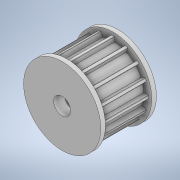
# Autodesk Inventor part: zahnrad2
Saved by Autodesk Inventor 2021 (Build 250183000, 183)
## iProperties
Created: 2021-08-20
Part Number: zahnrad2
Material: Generisch
Document SubType Name: Modeling
Designer: stroh
Density: 1 g/cm^3
Appearance: Vorgabe
Author: stroh
Autodesk Inventor part; units mm, degrees
ref_plane "YZ Plane" through (0, 0, 0) normal (1, 0, 0) x (0, 1, 0)
ref_plane "XZ Plane" through (0, 0, 0) normal (0, 1, 0) x (-1, 0, 0)
ref_plane "XY Plane" through (0, 0, 0) normal (0, 0, 1) x (1, 0, 0)
sketch "Skizze1" plane through (0, 0, 0) normal (0, 0, 1) x (1, 0, 0)
  circle A0 centre (0, 0) radius 9.99
  dimension "d0" = 19.98
  constraints: 1 centre point, 1 coincident
  measures "d0" diameter of A0
extrude "Extrusion1" add sketch "Skizze1" along normal blind 15
sketch "Skizze2" plane through (0, 0, 15) normal (0, 0, 1) x (1, 0, 0)
  circle A0 centre (0, 0) radius 9.99 projected
  line L0 (-0.5, 9.9775) -> (0.5, 9.9775)
  line L1 (-0.5, 9.9775) -> (-0.5177, 11.3774)
  line L2 (0.4823, 11.3774) -> (0.5, 9.9775)
  line L3 (-0.5177, 11.3774) -> (-0.419, 11.4786)
  line L4 (0.381, 11.4786) -> (0.4823, 11.3774)
  line L5 (-0.419, 11.4786) -> (0.381, 11.4786)
  line L6 (-4.2802, 9.0266) -> (-4.8322, 10.3132)
  line L7 (-4.8322, 10.3132) -> (-4.7798, 10.4445)
  line L8 (-4.7798, 10.4445) -> (-4.0407, 10.7507)
  line L9 (-4.0407, 10.7507) -> (-3.9084, 10.6959)
  line L10 (-3.9084, 10.6959) -> (-3.3563, 9.4093)
  line L11 (-4.2802, 9.0266) -> (-3.3563, 9.4093)
  line L12 (-7.4087, 6.7016) -> (-8.4111, 7.6789)
  line L13 (-8.4111, 7.6789) -> (-8.4129, 7.8203)
  line L14 (-8.4129, 7.8203) -> (-7.8472, 8.386)
  line L15 (-7.8472, 8.386) -> (-7.704, 8.386)
  line L16 (-7.704, 8.386) -> (-6.7016, 7.4087)
  line L17 (-7.4087, 6.7016) -> (-6.7016, 7.4087)
  line L18 (-9.4093, 3.3563) -> (-10.7094, 3.8756)
  line L19 (-10.7094, 3.8756) -> (-10.7652, 4.0056)
  line L20 (-10.7652, 4.0056) -> (-10.4591, 4.7447)
  line L21 (-10.4591, 4.7447) -> (-10.3268, 4.7995)
  line L22 (-10.3268, 4.7995) -> (-9.0266, 4.2802)
  line L23 (-9.4093, 3.3563) -> (-9.0266, 4.2802)
  line L24 (-9.9775, -0.5) -> (-11.3774, -0.5177)
  line L25 (-11.3774, -0.5177) -> (-11.4786, -0.419)
  line L26 (-11.4786, -0.419) -> (-11.4786, 0.381)
  line L27 (-11.4786, 0.381) -> (-11.3774, 0.4823)
  line L28 (-11.3774, 0.4823) -> (-9.9775, 0.5)
  line L29 (-9.9775, -0.5) -> (-9.9775, 0.5)
  line L30 (-9.0266, -4.2802) -> (-10.3132, -4.8322)
  line L31 (-10.3132, -4.8322) -> (-10.4445, -4.7798)
  line L32 (-10.4445, -4.7798) -> (-10.7507, -4.0407)
  line L33 (-10.7507, -4.0407) -> (-10.6959, -3.9084)
  line L34 (-10.6959, -3.9084) -> (-9.4093, -3.3563)
  line L35 (-9.0266, -4.2802) -> (-9.4093, -3.3563)
  line L36 (-6.7016, -7.4087) -> (-7.6789, -8.4111)
  line L37 (-7.6789, -8.4111) -> (-7.8203, -8.4129)
  line L38 (-7.8203, -8.4129) -> (-8.386, -7.8472)
  line L39 (-8.386, -7.8472) -> (-8.386, -7.704)
  line L40 (-8.386, -7.704) -> (-7.4087, -6.7016)
  line L41 (-6.7016, -7.4087) -> (-7.4087, -6.7016)
  line L42 (-3.3563, -9.4093) -> (-3.8756, -10.7094)
  line L43 (-3.8756, -10.7094) -> (-4.0056, -10.7652)
  line L44 (-4.0056, -10.7652) -> (-4.7447, -10.4591)
  line L45 (-4.7447, -10.4591) -> (-4.7995, -10.3268)
  line L46 (-4.7995, -10.3268) -> (-4.2802, -9.0266)
  line L47 (-3.3563, -9.4093) -> (-4.2802, -9.0266)
  line L48 (0.5, -9.9775) -> (0.5177, -11.3774)
  line L49 (0.5177, -11.3774) -> (0.419, -11.4786)
  line L50 (0.419, -11.4786) -> (-0.381, -11.4786)
  line L51 (-0.381, -11.4786) -> (-0.4823, -11.3774)
  line L52 (-0.4823, -11.3774) -> (-0.5, -9.9775)
  line L53 (0.5, -9.9775) -> (-0.5, -9.9775)
  line L54 (4.2802, -9.0266) -> (4.8322, -10.3132)
  line L55 (4.8322, -10.3132) -> (4.7798, -10.4445)
  line L56 (4.7798, -10.4445) -> (4.0407, -10.7507)
  line L57 (4.0407, -10.7507) -> (3.9084, -10.6959)
  line L58 (3.9084, -10.6959) -> (3.3563, -9.4093)
  line L59 (4.2802, -9.0266) -> (3.3563, -9.4093)
  line L60 (7.4087, -6.7016) -> (8.4111, -7.6789)
  line L61 (8.4111, -7.6789) -> (8.4129, -7.8203)
  line L62 (8.4129, -7.8203) -> (7.8472, -8.386)
  line L63 (7.8472, -8.386) -> (7.704, -8.386)
  line L64 (7.704, -8.386) -> (6.7016, -7.4087)
  line L65 (7.4087, -6.7016) -> (6.7016, -7.4087)
  line L66 (9.4093, -3.3563) -> (10.7094, -3.8756)
  line L67 (10.7094, -3.8756) -> (10.7652, -4.0056)
  line L68 (10.7652, -4.0056) -> (10.4591, -4.7447)
  line L69 (10.4591, -4.7447) -> (10.3268, -4.7995)
  line L70 (10.3268, -4.7995) -> (9.0266, -4.2802)
  line L71 (9.4093, -3.3563) -> (9.0266, -4.2802)
  line L72 (9.9775, 0.5) -> (11.3774, 0.5177)
  line L73 (11.3774, 0.5177) -> (11.4786, 0.419)
  line L74 (11.4786, 0.419) -> (11.4786, -0.381)
  line L75 (11.4786, -0.381) -> (11.3774, -0.4823)
  line L76 (11.3774, -0.4823) -> (9.9775, -0.5)
  line L77 (9.9775, 0.5) -> (9.9775, -0.5)
  line L78 (9.0266, 4.2802) -> (10.3132, 4.8322)
  line L79 (10.3132, 4.8322) -> (10.4445, 4.7798)
  line L80 (10.4445, 4.7798) -> (10.7507, 4.0407)
  line L81 (10.7507, 4.0407) -> (10.6959, 3.9084)
  line L82 (10.6959, 3.9084) -> (9.4093, 3.3563)
  line L83 (9.0266, 4.2802) -> (9.4093, 3.3563)
  line L84 (6.7016, 7.4087) -> (7.6789, 8.4111)
  line L85 (7.6789, 8.4111) -> (7.8203, 8.4129)
  line L86 (7.8203, 8.4129) -> (8.386, 7.8472)
  line L87 (8.386, 7.8472) -> (8.386, 7.704)
  line L88 (8.386, 7.704) -> (7.4087, 6.7016)
  line L89 (6.7016, 7.4087) -> (7.4087, 6.7016)
  line L90 (3.3563, 9.4093) -> (3.8756, 10.7094)
  line L91 (3.8756, 10.7094) -> (4.0056, 10.7652)
  line L92 (4.0056, 10.7652) -> (4.7447, 10.4591)
  line L93 (4.7447, 10.4591) -> (4.7995, 10.3268)
  line L94 (4.7995, 10.3268) -> (4.2802, 9.0266)
  line L95 (3.3563, 9.4093) -> (4.2802, 9.0266)
  dimension "d4" = 1
  dimension "d31" = 0.1
  dimension "d52" = 360
  constraints: 192 end point, 2 horizontal, 2 point on circle, 193 other
  measures "d4" distance of L0.start L0.end
  measures "d31" distance from line of L2 L4.start
extrude "Extrusion2" add sketch "Skizze2" against normal blind 15 contours A0 L72 L73 L74 L75 L76 | A0 L78 L79 L80 L81 L82 | L66 L67 L68 L69 L70 A0 | A0 L71 | A0 L84 L85 L86 L87 L88 | L60 L61 L62 L63 L64 A0 | A0 L65 | A0 L90 L91 L92 L93 L94 | L54 L55 L56 L57 L58 A0 | A0 L59 | L0 A0 | A0 L1 L3 L5 L4 L2 | L48 L49 L50 L51 L52 A0 | A0 L53 | A0 L6 L7 L8 L9 L10 | L42 L43 L44 L45 L46 A0 | A0 L12 L13 L14 L15 L16 | L36 L37 L38 L39 L40 A0 | L23 A0 | A0 L18 L19 L20 L21 L22 | L30 L31 L32 L33 L34 A0 | A0 L35 | L29 A0 | A0 L24 L25 L26 L27 L28
sketch "Skizze3" plane through (0, 0, 15) normal (0, 0, 1) x (1, 0, 0)
  circle A0 centre (0, 0) radius 12.5
  dimension "d15" = 25
  constraints: 1 centre point, 1 coincident
  measures "d15" diameter of A0
extrude "Extrusion3" add sketch "Skizze3" along normal blind 1.5
sketch "Skizze4" plane through (0, 0, 0) normal (0, 0, -1) x (-1, 0, 0)
  circle A0 centre (0, 0) radius 12.5
  dimension "d33" = 25
  constraints: 1 centre point, 1 coincident
  measures "d33" diameter of A0
extrude "Extrusion4" add sketch "Skizze4" along normal blind 1.5
sketch "Skizze5" plane through (0, 0, 16.5) normal (0, 0, 1) x (1, 0, 0)
  circle A0 centre (0, 0) radius 2.75
  dimension "d20" = 5.5
  constraints: 1 centre point, 1 coincident
  measures "d20" diameter of A0
extrude "Extrusion5" cut sketch "Skizze5" against normal blind 3.5
sketch "Skizze6" plane through (0, 0, -1.5) normal (0, 0, -1) x (-1, 0, 0)
  circle A0 centre (0, 0) radius 2.75
  dimension "d23" = 5.5
  constraints: 1 centre point, 1 coincident
  measures "d23" diameter of A0
extrude "Extrusion6" cut sketch "Skizze6" against normal blind 12
sketch "Skizze7" plane through (0, 0, 10.5) normal (0, 0, -1) x (-1, 0, 0)
  circle A0 centre (0, 0) radius 1.6
  dimension "d26" = 3.2
  constraints: 1 centre point, 1 coincident
  measures "d26" diameter of A0
extrude "Extrusion7" cut sketch "Skizze7" against normal blind 12
